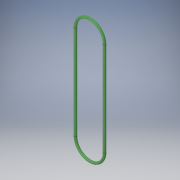
# Autodesk Inventor part: Polea
Saved by Autodesk Inventor 2019.4 (Build 234330000, 330)
## iProperties
Created: 2020-03-11
Part Number: Polea
Material: Genérico
Document SubType Name: Modeling
Designer: Usuario
Density: 1 g/cm^3
Appearance: Valor por defecto
Author: Usuario
Autodesk Inventor part; units mm, degrees
ref_plane "YZ Plane" through (0, 0, 0) normal (1, 0, 0) x (0, 1, 0)
ref_plane "XZ Plane" through (0, 0, 0) normal (0, 1, 0) x (-1, 0, 0)
ref_plane "XY Plane" through (0, 0, 0) normal (0, 0, 1) x (1, 0, 0)
sketch "Boceto1" plane through (0, 0, 0) normal (0, 0, 1) x (1, 0, 0)
  arc A0 (-28.75, 0) -> (28.75, 0) centre (0, 0) ccw
  arc A1 (28.75, 185.261) -> (-28.75, 185.261) centre (0, 185.261) ccw
  line L0 (-28.75, 185.261) -> (-28.75, 0)
  line L1 (28.75, 185.261) -> (28.75, 0)
  dimension "d0" = 185.261
  dimension "d1" = 57.5
  dimension "d2" = 57.5
  constraints: 4 end point, 4 point on circle, 4 tangent, 2 centre point, 1 coincident, 1 vertical alignment
  measures "d0" distance of point (0, 0) A1.centre
  measures "d1" diameter of A1
  measures "d2" diameter of A0
sketch "Boceto2" plane through (0, 0, 0) normal (0, 1, 0) x (-1, 0, 0)
  circle A0 centre (28.75, 0) radius 2.5
  point P0 (0, 0)
  dimension "d3" = 28.75
  dimension "d4" = 5
  constraints: 1 centre point, 1 horizontal alignment
  measures "d3" distance of point (0, 0) A0.centre
  measures "d4" diameter of A0
sweep "Barrido1" add profiles "Boceto2" path "Boceto1"
